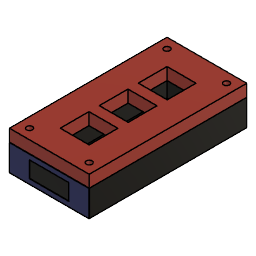
Hackpad Sai Shreyansh (Autodesk Fusion 360 design; units mm, degrees)
part number: 2026-07-27-19-25-03-228
Autodesk Fusion 360 part; units mm, degrees
sketch "Sketch4" plane through (0, 0, 0) normal (0, 0, 1) x (1, 0, 0)
  line L0 (0, 0) -> (19.4, 0)
  line L1 (19.4, 0) -> (19.4, 57.8)
  line L2 (19.4, 57.8) -> (0, 57.8)
  line L3 (0, 57.8) -> (0, 0)
  line L4 (-10, -10) -> (29.4, -10)
  line L5 (29.4, -10) -> (29.4, 67.8)
  line L6 (29.4, 67.8) -> (-10, 67.8)
  line L7 (-10, 67.8) -> (-10, -10)
  circle A0 centre (-5, -5) radius 1.45
  circle A1 centre (24.4, -5) radius 1.45
  circle A2 centre (-5, 62.8) radius 1.45
  circle A3 centre (24.4, 62.8) radius 1.45
extrude "Extrude3" add sketch "Sketch4" along normal blind 3 contours L4 L5 L6 L7 | A0 | A1 | A2 | A3 makes body 1
extrude "Extrude4" cut sketch "Sketch4" along normal blind 3 contours A0 | A1 | A2 | A3 bodies 1
extrude "Extrude5" add sketch "Sketch4" along normal blind 3 contours L0 L1 L2 L3 bodies 1
extrude "Extrude6" add sketch "Sketch4" along normal blind 10 from surface at 3 bodies 1
ref_plane "WorkPlane3" through (0, 0, 13) normal (0, 0, 1) x (1, 0, 0)
sketch "DXF_plate" plane through (0, 0, 13) normal (0, 0, 1) x (1, 0, 0)
  line L0 (-10, -10) -> (29.4, -10)
  line L1 (29.4, -10) -> (29.4, 67.8)
  line L2 (29.4, 67.8) -> (-10, 67.8)
  line L3 (-10, 67.8) -> (-10, -10)
  line L4 (2.5714, 41.087) -> (16.8286, 41.087)
  line L5 (16.8286, 41.087) -> (16.8286, 55.2463)
  line L6 (16.8286, 55.2463) -> (2.5714, 55.2463)
  line L7 (2.5714, 55.2463) -> (2.5714, 41.087)
  line L8 (2.5714, 21.8204) -> (16.8286, 21.8204)
  line L9 (16.8286, 21.8204) -> (16.8286, 35.9796)
  line L10 (16.8286, 35.9796) -> (2.5714, 35.9796)
  line L11 (2.5714, 35.9796) -> (2.5714, 21.8204)
  line L12 (2.5714, 2.5537) -> (16.8286, 2.5537)
  line L13 (16.8286, 2.5537) -> (16.8286, 16.7129)
  line L14 (16.8286, 16.7129) -> (2.5714, 16.7129)
  line L15 (2.5714, 16.7129) -> (2.5714, 2.5537)
  circle A0 centre (-5, -5) radius 1.45
  circle A1 centre (24.4, -5) radius 1.45
  circle A2 centre (-5, 62.8) radius 1.45
  circle A3 centre (24.4, 62.8) radius 1.45
extrude "Extrude9" add sketch "DXF_plate" along normal blind 3 contours L0 L1 L2 L3 | L4 L5 L6 L7 | L8 L9 L10 L11 | L12 L13 L14 L15 | A0 | A1 | A2 | A3 bodies 1
extrude "Extrude10" cut sketch "DXF_plate" along normal mid plane 6 contours L4 L5 L6 L7 | L8 L9 L10 L11 | L12 L13 L14 L15 bodies 1
extrude "Extrude11" cut sketch "DXF_plate" along normal mid plane 6 contours A0 | A1 | A2 | A3 bodies 1
ref_plane "WorkPlane4" through (0, 0, 16) normal (0, 0, 1) x (1, 0, 0)
sketch "DXF_plate_top" plane through (0, 0, 16) normal (0, 0, 1) x (1, 0, 0)
  line L0 (-10, -10) -> (29.4, -10)
  line L1 (29.4, -10) -> (29.4, 67.8)
  line L2 (29.4, 67.8) -> (-10, 67.8)
  line L3 (-10, 67.8) -> (-10, -10)
  line L4 (2.5714, 41.087) -> (16.8286, 41.087)
  line L5 (16.8286, 41.087) -> (16.8286, 55.2463)
  line L6 (16.8286, 55.2463) -> (2.5714, 55.2463)
  line L7 (2.5714, 55.2463) -> (2.5714, 41.087)
  line L8 (2.5714, 21.8204) -> (16.8286, 21.8204)
  line L9 (16.8286, 21.8204) -> (16.8286, 35.9796)
  line L10 (16.8286, 35.9796) -> (2.5714, 35.9796)
  line L11 (2.5714, 35.9796) -> (2.5714, 21.8204)
  line L12 (2.5714, 2.5537) -> (16.8286, 2.5537)
  line L13 (16.8286, 2.5537) -> (16.8286, 16.7129)
  line L14 (16.8286, 16.7129) -> (2.5714, 16.7129)
  line L15 (2.5714, 16.7129) -> (2.5714, 2.5537)
  circle A0 centre (-5, -5) radius 1.45
  circle A1 centre (24.4, -5) radius 1.45
  circle A2 centre (-5, 62.8) radius 1.45
  circle A3 centre (24.4, 62.8) radius 1.45
extrude "Extrude12" add sketch "DXF_plate_top" along normal blind 3 contours L0 L1 L2 L3 | L4 L5 L6 L7 | L8 L9 L10 L11 | L12 L13 L14 L15 | A0 | A1 | A2 | A3 bodies 1
extrude "Extrude13" cut sketch "DXF_plate_top" along normal mid plane 6 contours L4 L5 L6 L7 | L8 L9 L10 L11 | L12 L13 L14 L15 bodies 1
extrude "Extrude14" cut sketch "DXF_plate_top" along normal mid plane 6 contours A0 | A1 | A2 | A3 bodies 1
ref_plane "WorkPlane5" through (0, 0, 13) normal (0, 0, 1) x (1, 0, 0)
split "Split1" by plane through (0, 0, 13) normal (0, 0, 1) bodies 1 makes body 2 at (-3.2749, 26.5401, 19)
ref_plane "WorkPlane6" through (0, -10, 0) normal (0, 1, 0) x (0, 0, 1)
sketch "USB_cutout" plane through (0, -10, 0) normal (0, -1, 0) x (1, 0, 0)
  line L0 (29.4, 13) -> (-10, 13)
  line L1 (-10, 13) -> (-10, 0)
  line L2 (-10, 0) -> (29.4, 0)
  line L3 (29.4, 0) -> (29.4, 13)
  line L4 (0, 2.5) -> (19.4, 2.5)
  line L5 (19.4, 2.5) -> (19.4, 10.5)
  line L6 (19.4, 10.5) -> (0, 10.5)
  line L7 (0, 10.5) -> (0, 2.5)
extrude "Extrude17" add sketch "USB_cutout" along normal mid plane 0.2 separate body makes body 3
